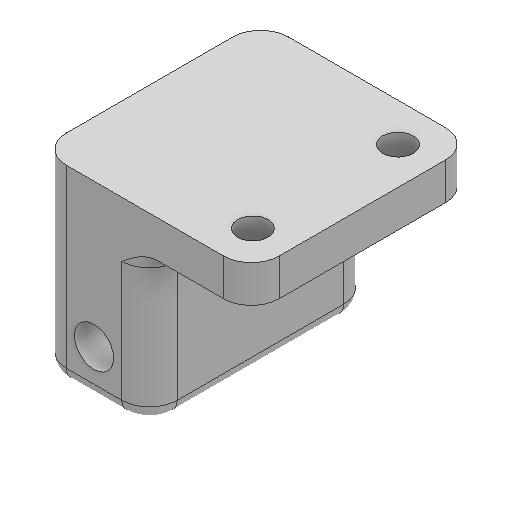
# Autodesk Inventor part: 3DP_ABS_PTFE_Tube_Stiffener
Saved by Autodesk Inventor 2026.1 (Build 301233000, 233)
## iProperties
Created: 2016-02-21
Part Number: 3DP_ABS_PTFE_Tube_Stiffener
Material: Ogólny
Document SubType Name: Modeling
Designer: Andrzej
Density: 1 g/cm^3
Appearance: Domyślna
Mass: 6.32166 g
Surface Area: 28.5046 cm^2
Volume: 6.32166 cm^3
Author: Andrzej
Autodesk Inventor part; units mm, degrees
ref_plane "YZ Plane" through (0, 0, 0) normal (1, 0, 0) x (0, 1, 0)
ref_plane "XZ Plane" through (0, 0, 0) normal (0, 1, 0) x (-1, 0, 0)
ref_plane "XY Plane" through (0, 0, 0) normal (0, 0, 1) x (1, 0, 0)
sketch "Szkic1" plane through (0, 0, 0) normal (0, 0, 1) x (1, 0, 0)
  line L0 (-5.5576, 4.7892) -> (17.4424, 4.7892)
  line L1 (17.4424, 4.7892) -> (17.4424, -19.2108)
  line L2 (17.4424, -19.2108) -> (-5.5576, -19.2108)
  line L3 (-5.5576, -19.2108) -> (-5.5576, 4.7892)
  line L4 (0.4424, -1.7194) -> (0.4424, -10.5168)
  line L5 (6.4424, 4.7892) -> (6.4424, -19.2108)
  circle A0 centre (13.4424, -15.0483) radius 3.1
  circle A1 centre (13.4424, 0.6267) radius 3.1
  point P0 (0, 0)
  dimension "d0" = 23
  dimension "d1" = 24
  dimension "d2" = 4
  dimension "d3" = 4
  dimension "d4" = 15.675
  dimension "d5" = 4.1625
  dimension "d6" = 13
  dimension "d7" = 12
  dimension "d19" = 6.2
  dimension "d20" = 6.2
  constraints: 12 end point, 2 centre point, 2 coincident, 2 parallel, 2 perpendicular, 2 point on line, 1 horizontal, 1 vertical
  measures "d0" distance of L1.end L2.end
  measures "d1" distance of L0.end L1.end
  measures "d2" distance from line of L1 point (13.442, 0.627)
  measures "d3" distance from line of L1 point (13.442, -15.048)
  measures "d4" distance of point (13.442, 0.627) point (13.442, -15.048)
  measures "d5" distance from line of L2 point (13.442, -15.048)
  measures "d6" distance from line of point (13.442, -15.048) L4
  measures "d7" distance between parallel lines of L3 L5
  measures "d19" diameter of A0
  measures "d20" diameter of A1
extrude "Wyciągnięcie proste1" add sketch "Szkic1" along normal blind 4 contours L0 L5 L2 L3 | L0 L1 L2 L5 | A0 | A1
extrude "Wyciągnięcie proste2" add sketch "Szkic1" against normal blind 16.5 contours L0 L5 L2 L3
hole "Otwór1" at (13.4424, 0.6267, 0) at (13.4424, -15.0483, 0) direction (0, 0, 1) diameter 3.3 end through all
extrude "Wyciągnięcie proste3" cut sketch "Szkic1" along normal blind 1.5 contours A0 | A1
sketch "Szkic2" plane through (-5.5576, 4.7892, 4) normal (0, 1, 0) x (1, 0, 0)
  line L0 (23, 4) -> (12, 4) projected
  line L1 (12, 4) -> (12, 20.5) projected
  line L2 (0, 20.5) -> (12, 20.5) projected
  line L3 (0, 0) -> (0, 20.5) projected
  line L4 (23, 0) -> (0, 0) projected
  line L5 (23, 4) -> (23, 0) projected
  point P0 (5.5576, 4)
  point P1 (6, 15.5)
  dimension "d23" = 15.5
  dimension "d24" = 12
  dimension "d25" = 6
  measures "d23" distance from line of point (6, 15.5) L4
  measures "d24" distance between parallel lines of L1 L3
  measures "d25" distance from line of L3 point (6, 15.5)
hole "Otwór2" at (0.4424, 4.7892, -11.5) direction (0, -1, 0) diameter 4.23 end through all
fillet "Zaokrąglenie1" radius 3 6 edges at (-5.5576, -19.2108, -6.25) (-5.5576, 4.7892, -6.25) (17.4424, 4.7892, 2) (17.4424, -19.2108, 2) (6.4424, 4.7892, -8.25) (6.4424, -19.2108, -8.25)
fillet "Zaokrąglenie2" radius 2 3 edges at (5.5637, 3.9105, 0) (5.5637, -18.3322, 0) (6.4424, -7.2108, 0)
fillet "Zaokrąglenie3" radius 1.5 8 edges at (5.5637, -18.3322, -16.5) (0.4424, -19.2108, -16.5) (-4.6789, -18.3322, -16.5) (-5.5576, -7.2108, -16.5) (-4.6789, 3.9105, -16.5) (0.4424, 4.7892, -16.5) (5.5637, 3.9105, -16.5) (6.4424, -7.2108, -16.5)
equation "\"d5\" = -0.5 * d4 + 0.5 * d1"
equation "\"d25\" = 0.5 * d24"
